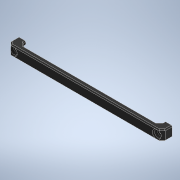
# Autodesk Inventor part: ModuleBracket_SLS
Saved by Autodesk Inventor 2021 (Build 250183000, 183)
## iProperties
Created: 2020-06-15
Part Number: ModuleBracket_SLS
Material: Generic
Document SubType Name: Modeling
Designer: Viktor Lindström
Density: 1 g/cm^3
Appearance: Default
Author: Viktor Lindström
## iProperties of the stored document _3DPrint.ipt
Created: 2020-06-18
Part Number: _3DPrint
Material: Generic
Document SubType Name: Modeling
Designer: Viktor Lindström
Density: 1 g/cm^3
Appearance: Default
Author: Viktor Lindström
Autodesk Inventor part; units mm, degrees
ref_plane "YZ Plane" through (0, 0, 0) normal (1, 0, 0) x (0, 1, 0)
ref_plane "XZ Plane" through (0, 0, 0) normal (0, 1, 0) x (-1, 0, 0)
ref_plane "XY Plane" through (0, 0, 0) normal (0, 0, 1) x (1, 0, 0)
sketch "Sketch1" plane through (0, 0, 0) normal (0, 0, 1) x (1, 0, 0)
  line L0 (-75, -5) -> (75, -5)
  line L1 (75, -5) -> (75, 5)
  line L2 (75, 5) -> (-75, 5)
  line L3 (-75, 5) -> (-75, -5)
  line L4 (-75, -5) -> (75, 5) construction
  line L5 (75, -5) -> (-75, 5) construction
  point P0 (0, 0)
  dimension "d0" = 150
  dimension "d1" = 10
  constraints: 12 end point, 2 midpoint, 2 parallel, 1 horizontal, 1 perpendicular
  measures "d0" distance of L1.end L2.end
  measures "d1" distance of L2.end L0.start
extrude "Extrusion1" add sketch "Sketch1" along normal mid plane 10
sketch "Sketch2" plane through (-75, -5, -5) normal (0, -1, 0) x (1, 0, 0)
  line L0 (150, 0) -> (0, 0) projected
  line L1 (7.5, 0) -> (142.5, 0)
  line L2 (142.5, 0) -> (142.5, 5)
  line L3 (142.5, 5) -> (7.5, 5)
  line L4 (7.5, 5) -> (7.5, 0)
  line L5 (150, 10) -> (150, 0) projected
  line L6 (0, 0) -> (0, 10) projected
  line L7 (0, 10) -> (150, 10) projected
  point P0 (75, 5)
  dimension "d7" = 67.5
  dimension "d8" = 135
  dimension "d9" = 5
  constraints: 8 end point, 2 parallel, 1 horizontal, 1 perpendicular, 2 other
  measures "d7" distance from line of point (75, 5) L4
  measures "d8" distance between parallel lines of L2 L4
  measures "d9" distance between parallel lines of L7 L3
extrude "Extrusion2" cut sketch "Sketch2" against normal through all contours L0 L4 L3 L2
sketch "Sketch3" plane through (67.5, -5, 0) normal (0, 0, -1) x (-1, 0, 0)
  line L0 (133, 5.8) -> (2, 5.8)
  line L1 (2, 5.8) -> (2, 4.2)
  line L2 (2, 4.2) -> (133, 4.2)
  line L3 (133, 4.2) -> (133, 5.8)
  line L4 (133, 5.8) -> (2, 4.2) construction
  line L5 (2, 5.8) -> (133, 4.2) construction
  line L6 (135, 10) -> (135, 0) projected
  point P0 (67.5, 5)
  point P1 (135, 5)
  dimension "d12" = 1.6
  dimension "d32" = 2
  constraints: 12 end point, 2 midpoint, 1 horizontal, 1 parallel, 1 perpendicular
  measures "d12" distance between parallel lines of L2 L0
  measures "d32" distance between parallel lines of L6 L3
extrude "Extrusion3" cut sketch "Sketch3" against normal blind 2
sketch "Sketch4" plane through (0, 0, -5) normal (0, 0, -1) x (-1, 0, 0)
  line L0 (105, 0) -> (-105, 0) projected
  line L1 (70, -3.4641) -> (67, -1.7321)
  line L2 (67, -1.7321) -> (67, 1.7321)
  line L3 (67, 1.7321) -> (70, 3.4641)
  line L4 (70, 3.4641) -> (73, 1.7321)
  line L5 (73, 1.7321) -> (73, -1.7321)
  line L6 (73, -1.7321) -> (70, -3.4641)
  point P0 (0, 0)
  point P1 (70, 0)
  point P2 (67, 0)
  dimension "d18" = 6
  dimension "d48" = 70
  constraints: 12 end point, 1 midpoint, 1 point on line, 13 other
  measures "d18" distance between parallel lines of L6 L3
  measures "d48" distance of point (0, 0) point (70, 0)
ref_plane "Work Plane1" through (67.5, -5, 0) normal (0, 0, -1) x (-1, 0, 0)
extrude "Extrusion5" cut sketch "Sketch4" against normal up to surface (5 mm away)
sketch "Sketch5" plane through (-67.5, -2.0207, 0) normal (0, 0, -1) x (1, 0, 0)
  line L0 (0, 2.9793) -> (0, 0) projected
  line L1 (-2.5, 1.4434) -> (0, 0) projected
  line L2 (-5.5, -0.2887) -> (-2.5, 1.4434) projected
  line L3 (-5.5, -3.7528) -> (-5.5, -0.2887) projected
  line L4 (-2.5, -5.4848) -> (-5.5, -3.7528) projected
  line L5 (0, -4.0415) -> (-2.5, -5.4848) projected
  line L6 (135, -7.0207) -> (0, -7.0207) projected
  line L7 (135, 2.9793) -> (135, -7.0207) projected
  line L8 (0, 2.9793) -> (135, 2.9793) projected
  line L9 (0, -4.0415) -> (0, -7.0207) projected
  line L10 (-37.5, -2.0207) -> (172.5, -2.0207) projected
  circle A0 centre (-2.5, -2.0207) radius 1.5
  point P0 (67.5, -2.0207)
  dimension "d25" = 5.5
  dimension "d33" = 3
  dimension "d34" = 3
  dimension "d35" = 6
  constraints: 1 centre point, 1 point on line
  measures "d25" distance between parallel lines of L3 L0
  measures "d33" diameter of A0
  measures "d34" distance from line of A0.centre L3
  measures "d35" distance between parallel lines of L2 L5
extrude "Extrusion6" cut sketch "Sketch5" against normal through all contours A0 L10 | L10 A0
sketch "Sketch6" plane through (0, 0, 5) normal (0, 0, 1) x (1, 0, 0)
  circle A0 centre (-70, 0) radius 3.25
  circle A1 centre (-70, 0) radius 1.5 projected
  line L0 (-105, 0) -> (105, 0) construction
  point P0 (0, 0)
  dimension "d70" = 6.5
  constraints: 1 centre point, 1 coincident, 1 concentric, 1 point on line
  measures "d70" diameter of A0
ref_plane "Work Plane2" through (-67.5, -2.0207, 2) normal (0, 0, -1) x (1, 0, 0)
extrude "Extrusion7" cut sketch "Sketch6" against normal blind 3.75 contours A0 | A1
mirror "Mirror1" about plane through (0, 0, 0) normal (1, 0, 0) of "Extrusion5", "Extrusion6", "Extrusion7"
chamfer "Chamfer3" distance 1 angle 45 6 edges at (75, 5, 0) (75, -5, 0) (-75, 5, 0) (-75, -5, 0) (0, 5, 5) (0, -5, 5)
chamfer "Chamfer5" distance 1 angle 45 2 edges at (73.25, 0, 5) (-73.25, 0, 5)
chamfer "Chamfer6" distance 3 angle 45 4 edges at (-67.5, 3.5104, 0) (-67.5, -3.5104, 0) (67.5, 3.5104, 0) (67.5, -3.5104, 0)
sketch "Sketch7" plane through (64.5, -5, 0) normal (0, 0, -1) x (-1, 0, 0)
  line L0 (132, 2.9793) -> (-3, 2.9793)
  line L1 (-3, 2.9793) -> (-3, 7.0207)
  line L2 (-3, 7.0207) -> (132, 7.0207)
  line L3 (132, 7.0207) -> (132, 2.9793)
  point P0 (64.5, 5)
  constraints: 8 end point, 2 parallel, 1 horizontal, 1 perpendicular
extrude "Extrusion8" cut sketch "Sketch7" along normal up to next
chamfer "Chamfer7" distance 1 angle 45 12 edges at (0, -0.8, 0) (0, 0.8, 0) (0, 5, 0) (-66, 5, -1.5) (-67.5, 5, -4) (-66, -5, -1.5) (-67.5, -5, -4) (0, -5, 0) (66, -5, -1.5) (67.5, -5, -4) (66, 5, -1.5) (67.5, 5, -4)
chamfer "Chamfer8" distance 0.5 angle 45 10 edges at (-73, 0, -5) (-71.5, -2.5981, -5) (-68.75, -2.7424, -5) (-71.5, 2.5981, -5) (-68.75, 2.7424, -5) (68.75, -2.7424, -5) (71.5, -2.5981, -5) (73, 0, -5) (71.5, 2.5981, -5) (68.75, 2.7424, -5)
thicken "Thicken1" operation add thickness 0.1 both sides no extend neighbours yes toward (0, -1, 0) faces at (21.8333, -0.8, 1.6667)
thicken "Thicken2" operation add thickness 0.1 both sides no extend neighbours yes toward (0, 1, 0) faces at (-21.8333, 0.8, 1.3333)
chamfer "Chamfer9" distance 3 angle 45 2 edges at (-75, 0, 5) (75, 0, 5)
chamfer "Chamfer10" distance 1 angle 45 4 edges at (73.5, 5, 3.5) (73.5, -5, 3.5) (-73.5, 5, 3.5) (-73.5, -5, 3.5)
ref_plane "Work Plane3" through (67.5, -2.0207, 2) normal (0, 0, 1) x (-1, 0, 0)
equation "\"d34\" = 0.5 * d35"
body "Solid1"
